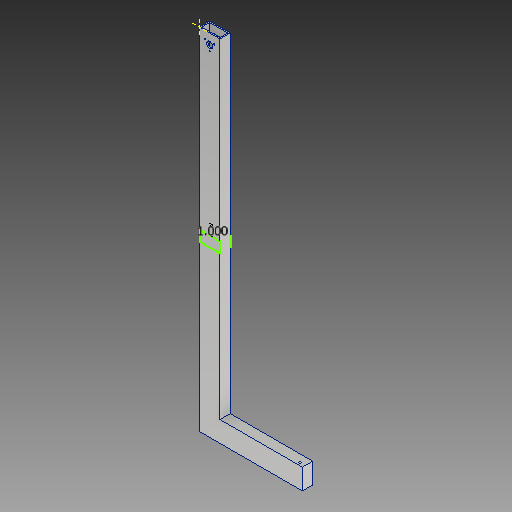
# Autodesk Inventor part: arm2v2
Saved by Autodesk Inventor 2017 (Build 210142000, 142)
## iProperties
Created: 2018-01-20
Part Number: arm2v2
Material: Aluminum 6061
Document SubType Name: Modeling
Designer: S331461152
Density: 2.7 g/cm^3
Appearance: Aluminum - Flat
Author: S331461152
Autodesk Inventor part; units mm, degrees
ref_plane "YZ Plane" through (0, 0, 0) normal (1, 0, 0) x (0, 1, 0)
ref_plane "XZ Plane" through (0, 0, 0) normal (0, 1, 0) x (-1, 0, 0)
ref_plane "XY Plane" through (0, 0, 0) normal (0, 0, 1) x (1, 0, 0)
sketch "Sketch1" plane through (0, 0, 0) normal (0, 0, 1) x (1, 0, 0)
  line L0 (0, 0) -> (0, -25.4)
  line L1 (0, -25.4) -> (50.8, -25.4)
  line L2 (50.8, -25.4) -> (50.8, 0)
  line L3 (50.8, 0) -> (0, 0)
  line L4 (0, -25.4) -> (1.524, -25.4)
  line L5 (3.048, -22.352) -> (47.752, -22.352)
  line L6 (50.8, -25.4) -> (23.876, -25.4)
  line L7 (47.752, -22.352) -> (47.752, -3.048)
  line L8 (50.8, 0) -> (50.8, -1.524)
  line L9 (47.752, -3.048) -> (3.048, -3.048)
  line L10 (0, 0) -> (1.524, 0)
  line L11 (3.048, -22.352) -> (3.048, -3.048)
  dimension "d53" = 25.4
  dimension "d54" = 50.8
  dimension "d55" = 3.048
  dimension "d56" = 3.048
  dimension "d57" = 3.048
  dimension "d58" = 3.048
  constraints: 24 end point, 5 perpendicular, 4 point on line, 1 vertical
  measures "d53" distance between parallel lines of L3 L1
  measures "d54" distance between parallel lines of L0 L2
  measures "d55" distance between parallel lines of L2 L7
  measures "d56" distance between parallel lines of L11 L0
  measures "d57" distance between parallel lines of L9 L3
  measures "d58" distance between parallel lines of L5 L1
extrude "Extrusion1" add sketch "Sketch1" along normal blind 812.8
sketch "Sketch2" plane through (50.8, -25.4, 0) normal (1, 0, 0) x (0, 0, -1)
  line L0 (-812.8, 25.4) -> (-812.8, 0) projected
  line L1 (-812.8, 25.4) -> (-863.6, 25.4)
  line L2 (-863.6, 25.4) -> (-863.6, 0)
  line L3 (-863.6, 0) -> (-812.8, 0)
  line L4 (0, 0) -> (-812.8, 0) projected
  line L5 (-812.8, 25.4) -> (-812.8, 0)
  line L6 (-812.8, 0) -> (-815.848, 0)
  line L7 (-815.848, 3.048) -> (-815.848, 47.752)
  line L8 (-812.8, 25.4) -> (-812.8, 22.352)
  line L9 (-815.848, 47.752) -> (-860.552, 47.752)
  line L10 (-863.6, 25.4) -> (-860.552, 25.4)
  line L11 (-863.6, 0) -> (-863.6, 3.048)
  line L12 (-860.552, 3.048) -> (-815.848, 3.048)
  line L13 (-860.552, 47.752) -> (-860.552, 3.048)
  point P0 (0, 25.4)
  constraints: 24 end point, 5 perpendicular, 4 point on line, 1 horizontal, 1 parallel, 1 vertical
extrude "Extrusion2" add sketch "Sketch2" against normal blind 254 contours L0 L3 L2 L1 L13 L12 L7 | L7 L12 L13 L1
sketch "Sketch3" plane through (0, -25.4, 0) normal (0, -1, 0) x (1, 0, 0)
  line L0 (0, 0) -> (50.8, 0) projected
  line L1 (50.8, 0) -> (0, 0)
  circle A0 centre (25.4, 25.4) radius 7.62
  circle A1 centre (25.4, 38.4302) radius 1.5875
  circle A2 centre (14.1155, 18.8849) radius 1.5875
  circle A3 centre (36.6845, 18.8849) radius 1.5875
  dimension "d23" = 360
  constraints: 4 centre point, 2 end point, 1 coincident, 1 horizontal, 7 other
extrude "Extrusion3" cut sketch "Sketch3" against normal blind 254
sketch "Sketch12" plane through (0, -25.4, 812.8) normal (0, 0, -1) x (-1, 0, 0)
  circle A0 centre (190.5, 6.35) radius 2.54
  line L0 (0, 25.4) -> (203.2, 25.4) projected
  line L1 (203.2, 25.4) -> (203.2, 0) projected
  dimension "d70" = 5.08
  dimension "d71" = 19.05
  dimension "d72" = 12.7
  constraints: 1 centre point
  measures "d70" diameter of A0
  measures "d71" distance from line of L0 A0.centre
  measures "d72" distance from line of L1 A0.centre
extrude "Extrusion10" cut sketch "Sketch12" against normal through all
sketch "Sketch13" plane through (0, -25.4, 0) normal (0, -1, 0) x (1, 0, 0)
  line L0 (50.8, 431.7892) -> (3.048, 431.7892)
  line L1 (0, 431.7892) -> (50.8, 431.7892)
  line L2 (50.8, 431.7892) -> (50.8, 457.1892)
  line L3 (50.8, 457.1892) -> (0, 457.1892)
  line L4 (0, 457.1892) -> (0, 431.7892)
  point P0 (50.8, 0)
  constraints: 10 end point, 1 perpendicular
sketch "Sketch14" plane through (0, 0, 0) normal (0, 1, 0) x (1, 0, 0)
  line L0 (50.8, -431.8) -> (0, -431.8)
  line L1 (50.8, -431.8) -> (50.8, -457.2)
  line L2 (50.8, -457.2) -> (0, -457.2)
  line L3 (0, -457.2) -> (0, -431.8)
  dimension "d78" = 25.4
  constraints: 8 end point, 1 horizontal, 1 perpendicular
  measures "d78" distance of L0.start L1.end
body "Solid1"
